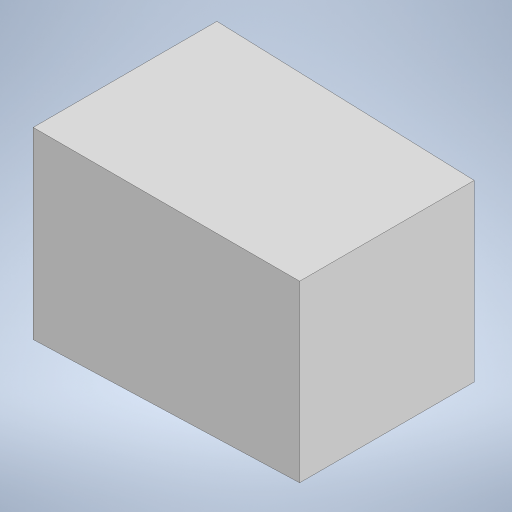
# Autodesk Inventor part: Piston Assembly Cast Image 2
Saved by Autodesk Inventor 2023 (Build 270158000, 158)
## iProperties
Created: 2022-12-28
Part Number: Piston Assembly Cast Image 2
Material: Generic
Document SubType Name: Modeling
Designer: tgr41
Density: 1 g/cm^3
Appearance: Default
Author: tgr41
Autodesk Inventor part; units mm, degrees
ref_plane "YZ Plane" through (0, 0, 0) normal (1, 0, 0) x (0, 1, 0)
ref_plane "XZ Plane" through (0, 0, 0) normal (0, 1, 0) x (-1, 0, 0)
ref_plane "XY Plane" through (0, 0, 0) normal (0, 0, 1) x (1, 0, 0)
sketch "Sketch2" plane through (0, 0, 0) normal (0, 1, 0) x (-1, 0, 0)
  line L0 (-25.4, 6.35) -> (-44.45, 6.35)
  line L1 (-44.45, 6.35) -> (-44.45, -6.35)
  line L2 (-44.45, -6.35) -> (-25.4, -6.35)
  line L3 (-25.4, -6.35) -> (-25.4, 6.35)
  line L4 (-25.4, 3.175) -> (-25.4, -3.175) projected
  point P0 (0, 0)
  point P1 (-25.4, 0)
  dimension "d6" = 0
  constraints: 8 end point, 2 parallel, 1 horizontal, 1 midpoint, 1 perpendicular
  measures "d6" distance between parallel lines of L3 L4
extrude "Extrusion1" add sketch "Sketch2" along normal mid plane 12.7
draft "FaceDraft1" angle 1 pull direction (1, 0, 0) faces at (31.75, -6.35, -2.1167) (38.1, 2.1167, 6.35) (38.1, -2.1167, -6.35) (31.75, 6.35, -2.1167) fixed edges at (44.45, -6.35, 0) (44.45, 0, 6.35) (44.45, 0, -6.35) (44.45, 6.35, 0)
body "Solid1"
